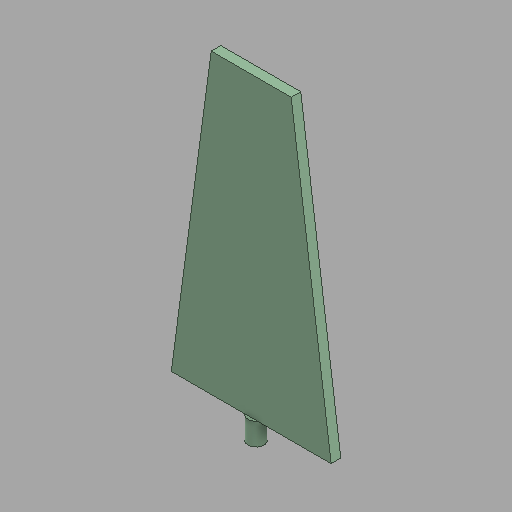
# Autodesk Inventor part: Антенна
Saved by Autodesk Inventor 2025 (Build 290162000, 162)
## iProperties
Created: 2024-11-27
Part Number: Антенна
Material: Типовые
Document SubType Name: Modeling
Designer: Artem Sannikov
Mass: 19 g
Surface Area: 78.8416 cm^2
Volume: 10.5999 cm^3
Density: 1.79246 g/cm^3
Appearance: Резина — зеленая
Author: Artem Sannikov
Autodesk Inventor part; units mm, degrees
ref_plane "YZ Plane" through (0, 0, 0) normal (1, 0, 0) x (0, 1, 0)
ref_plane "XZ Plane" through (0, 0, 0) normal (0, 1, 0) x (-1, 0, 0)
ref_plane "XY Plane" through (0, 0, 0) normal (0, 0, 1) x (1, 0, 0)
sketch "Эскиз1" plane through (0, 0, 0) normal (0, 1, 0) x (-1, 0, 0)
  circle A0 centre (0, 0) radius 2.5
  dimension "d0" = 5
  constraints: 1 centre point, 1 coincident
  measures "d0" diameter of A0
extrude "Выдавливание1" add sketch "Эскиз1" along normal blind 7
sketch "Эскиз2" plane through (0, 0, 0) normal (0, 0, 1) x (1, 0, 0)
  line L0 (2.5, 7) -> (-2.5, 7) projected
  line L1 (0, 7) -> (25, 7)
  line L2 (0, 7) -> (0, 100) construction
  line L3 (0, 100) -> (12.5, 100)
  line L4 (12.5, 100) -> (25, 7)
  line L5 (0, 7) -> (-25, 7)
  line L6 (0, 100) -> (-12.5, 100)
  line L7 (-12.5, 100) -> (-25, 7)
  point P0 (0, 0)
  dimension "d3" = 25
  dimension "d4" = 93
  constraints: 14 end point, 2 perpendicular, 2 symmetric about line, 1 collinear, 1 midpoint
  measures "d3" distance of L1.start L1.end
  measures "d4" distance of L1.start L2.end
extrude "Выдавливание2" add sketch "Эскиз2" along normal mid plane 3
